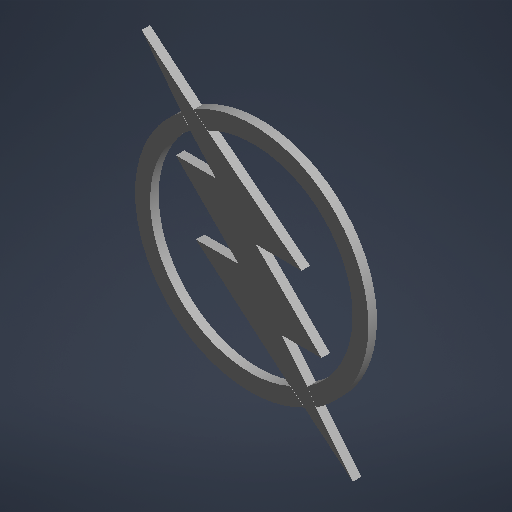
# Autodesk Inventor part: test_flash_cad_model
Saved by Autodesk Inventor 2026 (Build 300175050, 175E)
## iProperties
Part Number: test_flash_cad_model
Material: Generic
Document SubType Name: Modeling
Designer: Administrator
Appearance: Default
Author: Administrator
Autodesk Inventor part; units mm, degrees
ref_plane "Work Plane1" through (0, 0, 0) normal (0, 0, 1) x (1, 0, 0)
sketch "Sketch1" plane through (0, 0, 0) normal (0, 0, 1) x (1, 0, 0)
  line L0 (1.3, 10) -> (3.1, 8.5)
  line L1 (3.1, 8.5) -> (3.6, 8.1)
  line L2 (6.9, 5.5) -> (3.6, 8.1)
  line L3 (6.9, 5.5) -> (5.3, 5.5)
  line L4 (5.3, 5.5) -> (7.6, 3.2)
  line L5 (7.6, 3.2) -> (6.2, 3.2)
  line L6 (6.2, 3.2) -> (7.1, 2.1)
  line L7 (7.4, 1.6) -> (7.1, 2.1)
  line L8 (8.7, 0) -> (7.4, 1.6)
  line L9 (8.7, 0) -> (7, 1.4)
  line L10 (6.5, 1.8) -> (7, 1.4)
  line L11 (3.2, 4.6) -> (6.5, 1.8)
  line L12 (3.2, 4.6) -> (4.7, 4.6)
  line L13 (4.7, 4.6) -> (2.5, 6.8)
  line L14 (2.5, 6.8) -> (3.9, 6.8)
  line L15 (3.9, 6.8) -> (3, 7.8)
  line L16 (3, 7.8) -> (2.7, 8.2)
  line L17 (1.3, 10) -> (2.7, 8.2)
  constraints: 36 end point
extrude "Extrusion1" add sketch "Sketch1" along normal blind 0.3
ref_plane "Work Plane2" through (0, 0, 0) normal (0, 0, 1) x (1, 0, 0)
sketch "Sketch2" plane through (0, 0, 0) normal (0, 0, 1) x (1, 0, 0)
  line L0 (6.5, 1.8) -> (7, 1.4)
  arc A0 (2.7, 8.2) -> (7, 1.4) centre (5.106, 4.9619) ccw
  line L1 (3, 7.8) -> (2.7, 8.2)
  arc A1 (3, 7.8) -> (6.5, 1.8) centre (5.096, 5.0019) ccw
  constraints: 4 end point, 4 point on circle, 2 centre point
extrude "Extrusion2" add sketch "Sketch2" along normal blind 0.3 separate body
ref_plane "Work Plane3" through (0, 0, 0) normal (0, 0, 1) x (1, 0, 0)
sketch "Sketch3" plane through (0, 0, 0) normal (0, 0, 1) x (1, 0, 0)
  line L0 (3.1, 8.5) -> (3.6, 8.1)
  arc A0 (7.1, 2.1) -> (3.6, 8.1) centre (5.2133, 5.0203) ccw
  line L1 (7.4, 1.6) -> (7.1, 2.1)
  arc A1 (7.4, 1.6) -> (3.1, 8.5) centre (5.1775, 5.0048) ccw
  constraints: 4 end point, 4 point on circle, 2 centre point
extrude "Extrusion3" add sketch "Sketch3" along normal blind 0.3 separate body
body "Solid1"
body "Solid2"
body "Solid3"
